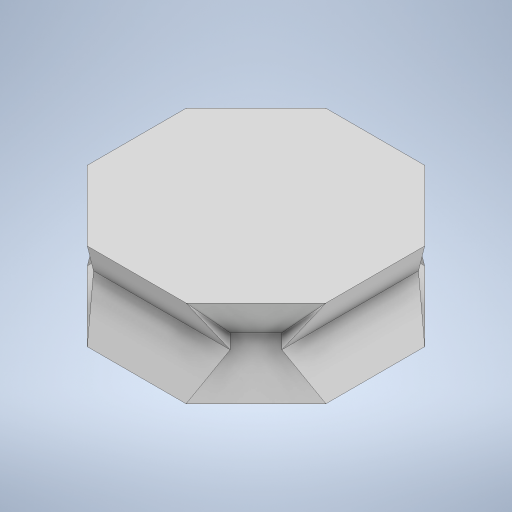
# Autodesk Inventor part: 팔각형 OV-PAM 층 한개
Saved by Autodesk Inventor 2024 (Build 280153000, 153)
## iProperties
Created: 2023-06-16
Part Number: 팔각형 OV-PAM 층 한개
Material: 일반
Document SubType Name: Modeling
Designer: jsw
Density: 1 g/cm^3
Appearance: 기본값
Mass: 73.6165 g
Surface Area: 139.388 cm^2
Volume: 73.6165 cm^3
Author: jsw
Autodesk Inventor part; units mm, degrees
ref_plane "YZ Plane" through (0, 0, 0) normal (1, 0, 0) x (0, 1, 0)
ref_plane "XZ Plane" through (0, 0, 0) normal (0, 1, 0) x (-1, 0, 0)
ref_plane "XY Plane" through (0, 0, 0) normal (0, 0, 1) x (1, 0, 0)
sketch "스케치1" plane through (0, 0, 0) normal (0, 1, 0) x (-1, 0, 0)
  line L0 (-32.5919, 13.5) -> (-13.5, 32.5919)
  line L1 (-13.5, 32.5919) -> (13.5, 32.5919)
  line L2 (13.5, 32.5919) -> (32.5919, 13.5)
  line L3 (32.5919, 13.5) -> (32.5919, -13.5)
  line L4 (32.5919, -13.5) -> (13.5, -32.5919)
  line L5 (13.5, -32.5919) -> (-13.5, -32.5919)
  line L6 (-13.5, -32.5919) -> (-32.5919, -13.5)
  line L7 (-32.5919, -13.5) -> (-32.5919, 13.5)
  line L8 (-13.8314, 33.3919) -> (13.8314, 33.3919)
  line L9 (13.8314, 33.3919) -> (33.3919, 13.8314)
  line L10 (33.3919, 13.8314) -> (33.3919, -13.8314)
  line L11 (33.3919, -13.8314) -> (13.8314, -33.3919)
  line L12 (13.8314, -33.3919) -> (-13.8314, -33.3919)
  line L13 (-13.8314, -33.3919) -> (-33.3919, -13.8314)
  line L14 (-33.3919, -13.8314) -> (-33.3919, 13.8314)
  line L15 (-33.3919, 13.8314) -> (-13.8314, 33.3919)
  point P0 (0, 0)
  point P1 (0, 0)
  point P2 (0, 0)
  dimension "d47" = 0.8
  dimension "d49" = 27
  constraints: 32 end point, 2 coincident, 2 horizontal, 34 other
  measures "d47" distance between parallel lines of L3 L10
  measures "d49" distance of L2.end L3.end
extrude "돌출2" add sketch "스케치1" along normal blind 12.21 contours L0 L1 L2 L3 L4 L5 L6 L7 | L8 L9 L10 L11 L12 L13 L14 L15
ref_plane "작업 평면2" through (33.3919, 0, 13.8314) normal (-0.8660254, -0.5, 0) x (0, 0, -1)
sketch "스케치3" plane through (33.3919, 0, 13.8314) normal (1, 0, 0) x (0, 0, -1)
  line L0 (0, 0) -> (0, 12.21) projected
  line L1 (0, 12.21) -> (27.6627, 12.21) projected
  line L2 (0, 0) -> (27.6627, 0)
  line L3 (27.6627, 0) -> (27.6627, 12.21)
  line L4 (27.6627, 12.21) -> (0, 12.21)
  line L5 (0, 12.21) -> (0, 0)
  line L6 (0, 12.21) -> (-7.244, 12.21)
  line L7 (-19.5605, 12.21) -> (0, 12.21) projected
  line L8 (0, 0) -> (-7.244, 12.21)
  line L9 (27.6627, 12.21) -> (34.9067, 12.21)
  line L10 (34.9067, 12.21) -> (27.6627, 0)
  point P0 (13.8314, 0)
  dimension "d17" = 120.68
  dimension "d18" = 120.68
  constraints: 16 end point, 2 parallel, 2 point on line, 1 horizontal, 1 perpendicular
  measures "d17" angle of L8 L2
  measures "d18" angle of L2 L10
extrude "돌출4" cut sketch "스케치3" against normal up to surface surface through (33.3919, 0, 13.8314) normal (-0.8660254, -0.5, 0)
sketch "스케치4" plane through (13.8314, 0, 33.3919) normal (0.7071068, 0, 0.7071068) x (0.7071068, 0, -0.7071068)
  line L0 (0, 0) -> (0, 12.21) projected
  line L1 (27.6627, 0) -> (27.6627, 12.21) projected
  line L2 (0, 0) -> (27.6627, 0)
  line L3 (27.6627, 0) -> (27.6627, 12.21)
  line L4 (27.6627, 12.21) -> (0, 12.21)
  line L5 (0, 12.21) -> (0, 0)
  line L6 (27.6627, 0) -> (17.6933, 12.21) projected
  line L7 (27.6627, 0) -> (18.9404, 12.21)
  line L8 (27.6627, 0) -> (0, 0) projected
  line L9 (0, 0) -> (8.7224, 12.21)
  line L10 (27.6627, 12.21) -> (0, 12.21) projected
  line L11 (13.8314, 12.21) -> (13.8314, 0)
  point P0 (8.7224, 12.21)
  point P1 (13.8314, 12.21)
  dimension "d41" = 10.218
  dimension "d42" = 5.109
  constraints: 14 end point, 2 midpoint, 2 parallel, 2 perpendicular, 2 point on line, 1 horizontal
  measures "d41" distance of L9.end L7.end
  measures "d42" distance of L7.end point (13.831, 12.21)
ref_plane "작업 평면3" through (13.8314, 0, 33.3919) normal (0.6123724, 0.5, 0.6123724) x (0.7071068, 0, -0.7071068)
extrude "돌출5" cut sketch "스케치4" against normal up to surface contours L9 L4 L11 L2 | L11 L4 L6 L2 | L6 L4 L7 surface through (13.8314, 0, 33.3919) normal (0.6123724, 0.5, 0.6123724)
pattern_circular "원형 패턴1" count 4 over 360 about axis through (0, -10, 0) along (0, 1, 0) of "돌출4"
pattern_circular "원형 패턴2" count 4 over 360 about axis through (0, -10, 0) along (0, 1, 0) of "돌출5"
mirror "미러5" about plane through (0, 12.21, 0) normal (0, 1, 0) of "돌출2", "돌출5", "원형 패턴2", "돌출4", "원형 패턴1"
ref_plane "작업 평면5" through (-13.8314, 12.21, -33.3919) normal (0, 1, 0) x (1, 0, 0)
equation "\"d42\" = 0.5 * d41"
